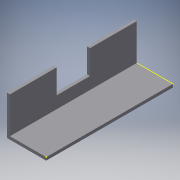
# Autodesk Inventor part: cut top wheel mout thingy
Saved by Autodesk Inventor 2017 (Build 210142000, 142)
## iProperties
Created: 2016-10-19
Part Number: cut top wheel mout thingy
Material: Generic
Document SubType Name: Modeling
Designer: Aditya
Density: 1 g/cm^3
Appearance: Default
Author: Aditya
Autodesk Inventor part; units mm, degrees
ref_plane "YZ Plane" through (0, 0, 0) normal (1, 0, 0) x (0, 1, 0)
ref_plane "XZ Plane" through (0, 0, 0) normal (0, 1, 0) x (-1, 0, 0)
ref_plane "XY Plane" through (0, 0, 0) normal (0, 0, 1) x (1, 0, 0)
sketch "Sketch1" plane through (0, 0, 0) normal (0, 1, 0) x (-1, 0, 0)
  line L0 (0, 0) -> (0, -133.35)
  line L1 (0, -133.35) -> (41.275, -133.35)
  line L2 (41.275, -133.35) -> (41.275, 0)
  line L3 (41.275, 0) -> (0, 0)
  dimension "d0" = 133.35
  dimension "d1" = 41.275
  constraints: 8 end point, 3 perpendicular, 1 vertical
  measures "d0" distance of L0.start L0.end
  measures "d1" distance of L0.end L1.end
extrude "Extrusion1" add sketch "Sketch1" along normal blind 3.175
sketch "Sketch2" plane through (0, 3.175, 0) normal (0, 1, 0) x (1, 0, 0)
  line L0 (-41.275, 133.35) -> (-41.275, 0) projected
  line L1 (-41.275, 0) -> (-38.1, 0)
  line L2 (-41.275, 0) -> (0, 0) projected
  line L3 (-38.1, 0) -> (-38.1, 133.35)
  line L4 (0, 133.35) -> (-41.275, 133.35) projected
  line L5 (-41.275, 133.35) -> (-41.275, 0)
  dimension "d4" = 3.175
  constraints: 6 end point, 2 point on line, 1 parallel, 1 perpendicular
  measures "d4" distance of L0.end L1.end
extrude "Extrusion2" add sketch "Sketch2" along normal blind 38.1
sketch "Sketch3" plane through (0, 41.275, 0) normal (0, 1, 0) x (1, 0, 0)
  line L0 (-41.275, 133.35) -> (-41.275, 0) projected
  line L1 (-41.275, 66.675) -> (-41.275, 84.1375)
  line L2 (-41.275, 66.675) -> (-41.275, 49.1998)
  line L3 (-41.275, 49.1998) -> (-38.1, 49.1998)
  line L4 (-38.1, 0) -> (-38.1, 133.35) projected
  line L5 (-38.1, 84.1375) -> (-41.275, 84.1375)
  line L6 (-38.1, 49.1998) -> (-38.1, 84.1375)
  point P0 (0, 0)
  dimension "d7" = 17.4625
  dimension "d8" = 17.4752
  constraints: 10 end point, 4 point on line, 1 collinear, 1 horizontal, 1 midpoint, 1 parallel
  measures "d7" distance of L1.start L1.end
  measures "d8" distance of L1.start L2.end
extrude "Extrusion3" cut sketch "Sketch3" against normal blind 25.4
sketch "Sketch4" plane through (0, 3.175, 0) normal (0, 1, 0) x (1, 0, 0)
  line L0 (0, 133.35) -> (-38.1, 133.35) projected
  point P0 (0, 0)
sketch "Sketch5" plane through (0, 3.175, 0) normal (0, 1, 0) x (1, 0, 0)
  line L0 (0, 0) -> (0, 133.35) projected
  line L1 (0, 66.675) -> (-38.3992, 66.675)
  line L2 (-19.1996, 66.675) -> (-19.1996, 118.0846)
  line L3 (-19.1996, 66.675) -> (-19.1996, 15.2654)
  circle A0 centre (-19.1996, 15.2654) radius 1.905
  circle A1 centre (-19.1996, 118.0846) radius 1.905
  dimension "d12" = 51.4096
  dimension "d13" = 51.4096
  dimension "d14" = 3.81
  dimension "d15" = 3.81
  constraints: 6 end point, 2 centre point, 2 coincident, 2 midpoint, 1 horizontal, 1 parallel, 1 vertical
  measures "d12" distance of L2.start L2.end
  measures "d13" distance of L2.start L3.end
  measures "d14" diameter of A0
  measures "d15" diameter of A1
extrude "Extrusion4" cut sketch "Sketch5" against normal blind 20.6375
body "Solid1"
